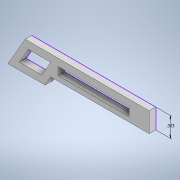
# Autodesk Inventor part: Crossbow Side
Saved by Autodesk Inventor 2021 (Build 250183000, 183)
## iProperties
Created: 2020-07-07
Part Number: Crossbow Side
Material: Generic
Document SubType Name: Modeling
Designer: saipr
Density: 1 g/cm^3
Appearance: Default
Author: saipr
Autodesk Inventor part; units mm, degrees
ref_plane "YZ Plane" through (0, 0, 0) normal (1, 0, 0) x (0, 1, 0)
ref_plane "XZ Plane" through (0, 0, 0) normal (0, 1, 0) x (-1, 0, 0)
ref_plane "XY Plane" through (0, 0, 0) normal (0, 0, 1) x (1, 0, 0)
sketch "Sketch1" plane through (0, 0, 0) normal (0, 0, 1) x (1, 0, 0)
  line L0 (0, 0) -> (3.4799, 6.0274)
  line L1 (3.4799, 6.0274) -> (12.1665, 6.0274)
  line L2 (0, 0) -> (8.6866, 0)
  line L3 (8.6866, 0) -> (12.1665, 6.0274)
  line L4 (-4.4376, -2.7527) -> (2.2208, 8.7801)
  line L5 (2.2208, 8.7801) -> (16.6041, 8.7801)
  line L6 (-4.4376, -2.7527) -> (9.9456, -2.7527)
  line L7 (9.9456, -2.7527) -> (12.1665, 1.0938)
  line L8 (12.1665, 1.0938) -> (50.2665, 1.0938)
  line L9 (50.2665, 1.0938) -> (50.2665, 8.7801)
  line L10 (50.2665, 8.7801) -> (12.1665, 8.7801)
  line L11 (15.0148, 6.0274) -> (42.492, 6.0274)
  line L12 (42.492, 6.0274) -> (42.492, 3.0137)
  line L13 (42.492, 3.0137) -> (15.0148, 3.0137)
  line L14 (15.0148, 3.0137) -> (15.0148, 6.0274)
  dimension "d26" = 7.6862
  constraints: 30 end point, 9 parallel, 2 point on line, 1 horizontal, 1 perpendicular
  measures "d26" distance of L8.end L9.end
extrude "Extrusion1" add sketch "Sketch1" along normal blind 2.54 contours L4 L5 L10 L9 L8 L7 L6 | L11 L12 L13 L14
extrude "Extrusion2" cut sketch "Sketch1" along normal blind 2.54 contours L11 L12 L13 L14
body "Solid1"
